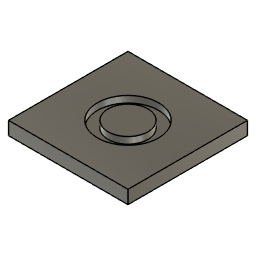
sand_cub_left (Autodesk Fusion 360 design; units mm, degrees)
Autodesk Fusion 360 part; units mm, degrees
note: some values were not read from the file. Set by a fixed rule: which sketch regions a step uses.
sketch "Sketch1" plane through (0, 0, 0) normal (0, 0, 1) x (1, 0, 0)
  line L0 (0, 0) -> (45, 0)
  line L1 (45, 0) -> (45, 45)
  line L2 (45, 45) -> (0, 45)
  line L3 (0, 45) -> (0, 0)
  dimension "d1" = 45
  dimension "d2" = 45
  constraint horizontal L0
  constraint vertical L1
  constraint horizontal L2
  constraint vertical L3
  constraint coincident L0.start L3.end
  measures "d1" distance of L0.start L0.end
  measures "d2" distance of L0.start L2.end
extrude "Extrude1" add sketch "Sketch1" along normal blind 5
sketch "Sketch2" plane through (0, 0, 5) normal (0, 0, 1) x (-1, 0, 0)
  line L0 (0, -45) -> (0, 0)
  line L1 (0, 0) -> (-45, 0)
  line L2 (-45, 0) -> (-45, -50)
  line L3 (-45, -45) -> (0, -45)
  line L4 (0, -45) -> (-45, -45)
  line L5 (-45, -45) -> (-45, -50)
  line L6 (-45, -50) -> (0, -50)
  line L7 (0, -50) -> (0, -45)
  line L8 (0, 0) -> (-45, 0)
  line L9 (-45, 0) -> (-45, 5)
  line L10 (-45, 5) -> (0, 5)
  line L11 (0, 5) -> (0, 0)
  line L12 (0, -50) -> (-45, 5)
  line L13 (-45, -50) -> (0, 5)
  circle A0 centre (-22.5, -22.5) radius 7.5
  circle A1 centre (-22.5, -22.5) radius 11.5
  dimension "d5" = 45
  dimension "d6" = 5
  dimension "d7" = 45
  dimension "d8" = 5
  dimension "d13" = 15
  dimension "d14" = 23
  constraint horizontal L4
  constraint vertical L5
  constraint horizontal L6
  constraint vertical L7
  constraint coincident L0.start L3.end
  constraint horizontal L8
  constraint vertical L9
  constraint horizontal L10
  constraint vertical L11
  constraint coincident L0.end L1.start
  constraint midpoint L13 A0.centre
  constraint concentric A0 A1
  measures "d5" distance of L0.start L3.start
  measures "d6" distance of L0.start L6.end
  measures "d7" distance of L0.end L1.end
  measures "d8" distance of L0.end L10.end
  measures "d13" diameter of A0
  measures "d14" diameter of A1
extrude "Extrude3" cut sketch "Sketch2" against normal blind 2.5 contours L12 L13 A0 A1 | L12 L13 A0 A1 | L12 L13 A0 A1 | L12 L13 A0 A1
